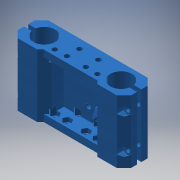
# Autodesk Inventor part: ChimeraXCarriage6
Saved by Autodesk Inventor 2016 (Build 200138000, 138)
## iProperties
Category: Print
Created: 2015-03-10
Part Number: ChimeraXCarriage6
Material: ABS Plastic
Document SubType Name: Modeling
Designer: Jack
Density: 1.06 g/cm^3
Appearance: Cyan
Mass: 40.4192 g
Surface Area: 204.208 cm^2
Volume: 38.1313 cm^3
Author: Jack
Title: Chimera X Carriage V6
Autodesk Inventor part; units mm, degrees
ref_plane "YZ Plane" through (0, 0, 0) normal (1, 0, 0) x (0, 1, 0)
ref_plane "XZ Plane" through (0, 0, 0) normal (0, 1, 0) x (-1, 0, 0)
ref_plane "XY Plane" through (0, 0, 0) normal (0, 0, 1) x (1, 0, 0)
sketch "Sketch1" plane through (0, 0, 0) normal (0, 0, 1) x (1, 0, 0)
  arc A0 (-7.6035, -1.5) -> (-7.6035, 1.5) centre (0, 0) ccw
  arc A1 (62.6035, 1.5) -> (62.6035, -1.5) centre (55, 0) ccw
  line L0 (-7.6035, -1.5) -> (-13, -1.5)
  line L1 (-13, -1.5) -> (-13, -11)
  line L2 (-13, -11) -> (11, -11)
  line L3 (11, -11) -> (11, 3)
  line L4 (11, 3) -> (44, 3)
  line L5 (44, 3) -> (44, -11)
  line L6 (44, -11) -> (68, -11)
  line L7 (68, -11) -> (68, -1.5)
  line L8 (68, -1.5) -> (62.6035, -1.5)
  line L9 (62.6035, 1.5) -> (68, 1.5)
  line L10 (68, 1.5) -> (68, 11)
  line L11 (68, 11) -> (44, 11)
  line L12 (44, 11) -> (44, 11)
  line L13 (44, 11) -> (11, 11)
  line L14 (11, 11) -> (11, 11)
  line L15 (11, 11) -> (-13, 11)
  line L16 (-13, 11) -> (-13, 1.5)
  line L17 (-13, 1.5) -> (-7.6035, 1.5)
  dimension "d0" = 15.5
  dimension "d1" = 55
  dimension "d2" = 1.5
  dimension "d3" = 13
  dimension "d4" = 11
  dimension "d5" = 11
  dimension "d6" = 11
  dimension "d7" = 13
  dimension "d8" = 14
  dimension "d9" = 8
  constraints: 36 end point, 12 perpendicular, 6 point on line, 4 equal length, 4 point on circle, 4 vertical alignment, 2 centre point, 1 coincident, 1 equal radius, 1 horizontal, 1 horizontal alignment, 1 parallel, 1 vertical
  measures "d0" diameter of A0
  measures "d1" distance of A1.centre point (0, 0)
  measures "d2" distance from line of point (0, 0) L0
  measures "d3" distance from line of point (0, 0) L16
  measures "d4" distance from line of L15 point (0, 0)
  measures "d5" distance from line of L14 point (0, 0)
  measures "d6" distance from line of L2 point (0, 0)
  measures "d7" distance from line of A1.centre L10
  measures "d8" distance of L2.end L3.end
  measures "d9" distance between parallel lines of L4 L13
extrude "Extrusion1" add sketch "Sketch1" along normal blind 45
chamfer "Chamfer1" distance 5 angle 45 6 edges at (-13, 11, 22.5) (-13, -11, 22.5) (68, -11, 22.5) (68, 11, 22.5) (44, -11, 22.5) (11, -11, 22.5)
sketch "Sketch2" plane through (-8, 11, 0) normal (0, 1, 0) x (1, 0, 0)
  line L0 (71, 0) -> (71, -45) projected
  line L1 (0, -45) -> (0, 0) projected
  line L2 (76, -45) -> (76, 0) projected
  line L3 (-5, 0) -> (-5, -45) projected
  line L4 (76, 0) -> (71, 0) projected
  line L5 (71, -45) -> (76, -45) projected
  point P0 (8, 0)
  point P1 (-2.5, -10)
  point P2 (-2.5, -35)
  point P3 (73.5, -10)
  point P4 (73.5, -35)
  dimension "d18" = 2.5
  dimension "d19" = 2.5
  dimension "d20" = 10
  dimension "d21" = 10
  constraints: 2 horizontal alignment, 2 vertical alignment
  measures "d18" distance from line of L1 point (-2.5, -10)
  measures "d19" distance from line of L0 point (73.5, -10)
  measures "d20" distance from line of L4 point (73.5, -10)
  measures "d21" distance from line of L5 point (73.5, -35)
hole "Hole1" at (-10.5, 11, 10) at (-10.5, 11, 35) at (65.5, 11, 10) at (65.5, 11, 35) direction (0, -1, 0) diameter 3.5 end through all counterbore diameter 7.3 counterbore depth 5
sketch "Sketch3" plane through (49, -11, 0) normal (0, -1, 0) x (1, 0, 0)
  circle A0 centre (16.5, 10) radius 1.75 projected
  circle A1 centre (16.5, 35) radius 1.75 projected
  circle A2 centre (-59.5, 35) radius 1.75 projected
  circle A3 centre (-59.5, 10) radius 1.75 projected
  line L0 (16.5, 13.1754) -> (19.25, 11.5877)
  line L1 (19.25, 11.5877) -> (19.25, 8.4123)
  line L2 (19.25, 8.4123) -> (16.5, 6.8246)
  line L3 (16.5, 6.8246) -> (13.75, 8.4123)
  line L4 (13.75, 8.4123) -> (13.75, 11.5877)
  line L5 (13.75, 11.5877) -> (16.5, 13.1754)
  line L6 (16.5, 31.8246) -> (13.75, 33.4123)
  line L7 (13.75, 33.4123) -> (13.75, 36.5877)
  line L8 (13.75, 36.5877) -> (16.5, 38.1754)
  line L9 (16.5, 38.1754) -> (19.25, 36.5877)
  line L10 (19.25, 36.5877) -> (19.25, 33.4123)
  line L11 (19.25, 33.4123) -> (16.5, 31.8246)
  circle A4 centre (-59.5, 10) radius 1.75 projected
  line L12 (-59.5, 6.8246) -> (-62.25, 8.4123)
  line L13 (-62.25, 8.4123) -> (-62.25, 11.5877)
  line L14 (-62.25, 11.5877) -> (-59.5, 13.1754)
  line L15 (-59.5, 13.1754) -> (-56.75, 11.5877)
  line L16 (-56.75, 11.5877) -> (-56.75, 8.4123)
  line L17 (-56.75, 8.4123) -> (-59.5, 6.8246)
  line L18 (-59.5, 38.1754) -> (-56.75, 36.5877)
  line L19 (-56.75, 36.5877) -> (-56.75, 33.4123)
  line L20 (-56.75, 33.4123) -> (-59.5, 31.8246)
  line L21 (-59.5, 31.8246) -> (-62.25, 33.4123)
  line L22 (-62.25, 33.4123) -> (-62.25, 36.5877)
  line L23 (-62.25, 36.5877) -> (-59.5, 38.1754)
  point P0 (-49, 0)
  dimension "d29" = 5.5
  constraints: 48 end point, 4 coincident, 4 vertical, 3 parallel, 52 other
  measures "d29" distance between parallel lines of L4 L1
extrude "Extrusion2" cut sketch "Sketch3" against normal blind 5
sketch "Sketch5" plane through (-8, 11, 0) normal (0, 1, 0) x (1, 0, 0)
  line L0 (0, 0) -> (71, 0) projected
  line L1 (52, 0) -> (52, -45) projected
  point P0 (8, 0)
  point P1 (48.5, -22.5)
  point P2 (36.5, -31)
  point P3 (36.5, -14)
  dimension "d44" = 17
  dimension "d45" = 12
  dimension "d46" = 3.5
  dimension "d47" = 22.5
  dimension "d48" = 8.5
  constraints: 1 vertical alignment
  measures "d44" distance of point (36.5, -31) point (36.5, -14)
  measures "d45" horizontal distance of point (36.5, -14) point (48.5, -22.5)
  measures "d46" distance from line of L1 point (48.5, -22.5)
  measures "d47" distance from line of L0 point (48.5, -22.5)
  measures "d48" vertical distance of point (48.5, -22.5) point (36.5, -31)
hole "Hole3" at (40.5, 11, 22.5) at (28.5, 11, 31) at (28.5, 11, 14) direction (0, -1, 0) diameter 3.5 end through all counterbore diameter 7.3 counterbore depth 3.5
sketch "Sketch6" plane through (-8, 11, 0) normal (0, 1, 0) x (1, 0, 0)
  circle A0 centre (48.5, -22.5) radius 3.65 projected
  arc A1 (51.9105, -7.1631) -> (49.5, -4) centre (49.5, -6.5) ccw
  arc A2 (49.5, -41) -> (51.9105, -37.8369) centre (49.5, -38.5) ccw
  arc A3 (49.8388, -30.3064) -> (41.1612, -30.3064) centre (45.5, -31.5) ccw
  arc A4 (41.1612, -14.6936) -> (49.8388, -14.6936) centre (45.5, -13.5) ccw
  arc A5 (41.5, -4) -> (39.0895, -7.1631) centre (41.5, -6.5) ccw
  arc A6 (39.0895, -37.8369) -> (41.5, -41) centre (41.5, -38.5) ccw
  line L0 (41.5, -4) -> (49.5, -4)
  line L1 (51.9105, -7.1631) -> (49.8388, -14.6936)
  line L2 (39.0895, -7.1631) -> (41.1612, -14.6936)
  line L3 (49.8388, -30.3064) -> (51.9105, -37.8369)
  line L4 (41.1612, -30.3064) -> (39.0895, -37.8369)
  line L5 (41.5, -41) -> (49.5, -41)
  point P0 (8, 0)
  dimension "d136" = 9
  dimension "d138" = 4
  dimension "d139" = 9
  dimension "d140" = 9
  dimension "d141" = 18
  dimension "d142" = 3
  dimension "d143" = 7
  dimension "d144" = 7
  dimension "d145" = 5
  dimension "d146" = 4
  constraints: 12 end point, 12 point on circle, 12 tangent, 6 centre point, 3 equal radius, 3 vertical alignment, 2 horizontal alignment, 1 horizontal
  measures "d136" diameter of A3
  measures "d138" horizontal distance of A2.centre A3.centre
  measures "d139" vertical distance of A0.centre A3.centre
  measures "d140" diameter of A4
  measures "d141" distance of A3.centre A4.centre
  measures "d142" horizontal distance of A0.centre A4.centre
  measures "d143" vertical distance of A2.centre A3.centre
  measures "d144" vertical distance of A4.centre A1.centre
  measures "d145" diameter of A1
  measures "d146" horizontal distance of A4.centre A5.centre
extrude "Extrusion3" cut sketch "Sketch6" against normal up to surface (8 mm away) contours L1 A4 L2 A5 L0 A1 | L5 A6 L4 A3 L3 A2
sketch "Sketch7" plane through (0, 0, 45) normal (0, 0, 1) x (1, 0, 0)
  line L0 (11, -6) -> (6, -11) projected
  line L1 (11, -6) -> (11, 3) projected
  line L2 (11, 3) -> (44, 3) projected
  line L3 (44, 3) -> (44, -6) projected
  arc A0 (62.6035, 1.5) -> (62.6035, -1.5) centre (55, 0) ccw projected
  line L4 (8.3, -8.7) -> (46.7, -8.7)
  line L5 (44, -6) -> (49, -11) projected
  dimension "d66" = 8.7
  constraints: 2 end point, 2 point on line, 1 horizontal
  measures "d66" distance from line of A0.centre L4
extrude "Extrusion4" add sketch "Sketch7" against normal blind 5
sketch "Sketch8" plane through (0, 0, 0) normal (0, 0, -1) x (-1, 0, 0)
  line L0 (-11, -6) -> (-8.3, -8.7) projected
  line L1 (-11, 3) -> (-11, -6) projected
  line L2 (-31.5, 3) -> (-11, 3) projected
  line L3 (-44, -6) -> (-44, 3) projected
  line L4 (-46.7, -8.7) -> (-44, -6) projected
  line L5 (-46.7, -8.7) -> (-8.3, -8.7) projected
  line L6 (-31.5, 3) -> (-43.5, 3) projected
  line L7 (-44, 3) -> (-43.5, 3) projected
extrude "Extrusion5" add sketch "Sketch8" against normal blind 5
sketch "Sketch9" plane through (0, 0, 0) normal (0, 0, -1) x (-1, 0, 0)
  arc A0 (7.6035, 1.5) -> (7.6035, -1.5) centre (0, 0) ccw projected
  line L0 (13, 1.5) -> (13, 6) projected
  circle A1 centre (-34.25, 4.45) radius 1.75
  circle A2 centre (-34.25, -4.45) radius 1.75
  circle A3 centre (-20.75, 4.45) radius 1.75
  circle A4 centre (-20.75, -4.45) radius 1.75
  dimension "d71" = 3.5
  dimension "d72" = 13.5
  dimension "d73" = 8.9
  dimension "d74" = 4.45
  dimension "d76" = 33.75
  constraints: 4 centre point, 3 equal radius, 2 horizontal alignment, 2 vertical alignment
  measures "d71" diameter of A1
  measures "d72" distance of A3.centre A1.centre
  measures "d73" distance of A3.centre A4.centre
  measures "d74" vertical distance of A0.centre A3.centre
  measures "d76" distance from line of L0 A3.centre
extrude "Extrusion6" cut sketch "Sketch9" against normal up to surface (5 mm away)
sketch "Sketch10" plane through (0, 0, 45) normal (0, 0, 1) x (1, 0, 0)
  circle A0 centre (34.25, -4.45) radius 1.75 projected
  circle A1 centre (20.75, -4.45) radius 1.75 projected
  arc A2 (19.7702, 3) -> (21.7298, 3) centre (20.75, 4.45) ccw projected
  arc A3 (33.2702, 3) -> (35.2298, 3) centre (34.25, 4.45) ccw projected
  circle A4 centre (20.75, 4.45) radius 1.75 projected
  circle A5 centre (34.25, 4.45) radius 1.75 projected
extrude "Extrusion7" cut sketch "Sketch10" against normal up to surface (5 mm away)
sketch "Sketch11" plane through (0, 0, 40) normal (0, 0, -1) x (-1, 0, 0)
  arc A0 (-21.7298, 3) -> (-19.7702, 3) centre (-20.75, 4.45) ccw projected
  arc A1 (-35.2298, 3) -> (-33.2702, 3) centre (-34.25, 4.45) ccw projected
  circle A2 centre (-20.75, -4.45) radius 1.75 projected
  circle A3 centre (-34.25, -4.45) radius 1.75 projected
  line L0 (-31.0746, 4.45) -> (-32.6623, 1.7)
  line L1 (-32.6623, 1.7) -> (-35.8377, 1.7)
  line L2 (-35.8377, 1.7) -> (-37.4254, 4.45)
  line L3 (-37.4254, 4.45) -> (-35.8377, 7.2)
  line L4 (-35.8377, 7.2) -> (-32.6623, 7.2)
  line L5 (-32.6623, 7.2) -> (-31.0746, 4.45)
  line L6 (-31.0746, -4.45) -> (-32.6623, -7.2)
  line L7 (-32.6623, -7.2) -> (-35.8377, -7.2)
  line L8 (-35.8377, -7.2) -> (-37.4254, -4.45)
  line L9 (-37.4254, -4.45) -> (-35.8377, -1.7)
  line L10 (-35.8377, -1.7) -> (-32.6623, -1.7)
  line L11 (-32.6623, -1.7) -> (-31.0746, -4.45)
  line L12 (-23.9254, -4.45) -> (-22.3377, -1.7)
  line L13 (-22.3377, -1.7) -> (-19.1623, -1.7)
  line L14 (-19.1623, -1.7) -> (-17.5746, -4.45)
  line L15 (-17.5746, -4.45) -> (-19.1623, -7.2)
  line L16 (-19.1623, -7.2) -> (-22.3377, -7.2)
  line L17 (-22.3377, -7.2) -> (-23.9254, -4.45)
  line L18 (-23.9254, 4.45) -> (-22.3377, 7.2)
  line L19 (-22.3377, 7.2) -> (-19.1623, 7.2)
  line L20 (-19.1623, 7.2) -> (-17.5746, 4.45)
  line L21 (-17.5746, 4.45) -> (-19.1623, 1.7)
  line L22 (-19.1623, 1.7) -> (-22.3377, 1.7)
  line L23 (-22.3377, 1.7) -> (-23.9254, 4.45)
  point P0 (0, 0)
  dimension "d81" = 5.5
  constraints: 48 end point, 4 coincident, 4 horizontal, 3 equal length, 52 other
  measures "d81" distance between parallel lines of L8 L11
extrude "Extrusion8" cut sketch "Sketch11" along normal blind 3.5 and the other way blind 3
sketch "Sketch12" plane through (0, 0, 5) normal (0, 0, 1) x (1, 0, 0)
  circle A0 centre (34.25, 4.45) radius 1.75 projected
  line L0 (31.0746, 4.45) -> (32.6623, 1.7) projected
  line L1 (32.6623, 7.2) -> (31.0746, 4.45) projected
  line L2 (35.8377, 7.2) -> (32.6623, 7.2) projected
  line L3 (37.4254, 4.45) -> (35.8377, 7.2) projected
  line L4 (35.8377, 1.7) -> (37.4254, 4.45) projected
  line L5 (32.6623, 1.7) -> (35.8377, 1.7) projected
  circle A1 centre (34.25, -4.45) radius 1.75 projected
  line L6 (31.0746, -4.45) -> (32.6623, -7.2) projected
  line L7 (32.6623, -1.7) -> (31.0746, -4.45) projected
  line L8 (35.8377, -1.7) -> (32.6623, -1.7) projected
  line L9 (37.4254, -4.45) -> (35.8377, -1.7) projected
  line L10 (35.8377, -7.2) -> (37.4254, -4.45) projected
  line L11 (32.6623, -7.2) -> (35.8377, -7.2) projected
  circle A2 centre (20.75, 4.45) radius 1.75 projected
  line L12 (23.9254, 4.45) -> (22.3377, 7.2) projected
  line L13 (22.3377, 1.7) -> (23.9254, 4.45) projected
  line L14 (19.1623, 1.7) -> (22.3377, 1.7) projected
  line L15 (17.5746, 4.45) -> (19.1623, 1.7) projected
  line L16 (19.1623, 7.2) -> (17.5746, 4.45) projected
  line L17 (22.3377, 7.2) -> (19.1623, 7.2) projected
  circle A3 centre (20.75, -4.45) radius 1.75 projected
  line L18 (23.9254, -4.45) -> (22.3377, -1.7) projected
  line L19 (22.3377, -7.2) -> (23.9254, -4.45) projected
  line L20 (19.1623, -7.2) -> (22.3377, -7.2) projected
  line L21 (17.5746, -4.45) -> (19.1623, -7.2) projected
  line L22 (19.1623, -1.7) -> (17.5746, -4.45) projected
  line L23 (22.3377, -1.7) -> (19.1623, -1.7) projected
  point P0 (0, 0)
extrude "Extrusion9" cut sketch "Sketch12" along normal blind 3.5 and the other way blind 3 contours A0 | L1 L2 L3 L4 L5 L0 | A1 | L7 L8 L9 L10 L11 L6 | A2 | L13 L14 L15 L16 L17 L12 | A3 | L19 L20 L21 L22 L23 L18
ref_plane "Work Plane1" through (0, 0, 2) normal (0, 0, -1) x (-1, 0, 0)
sketch "Sketch15" plane through (0, 0, 2) normal (0, 0, -1) x (-1, 0, 0)
  circle A0 centre (-20.75, 4.45) radius 1.75 projected
  circle A1 centre (-20.75, -4.45) radius 1.75 projected
  circle A2 centre (-34.25, -4.45) radius 1.75 projected
  circle A3 centre (-34.25, 4.45) radius 1.75 projected
  line L0 (-6, -11) -> (-8.3, -8.7) projected
  line L1 (-6, -11) -> (8, -11) projected
  line L2 (13, -6) -> (8, -11) projected
  line L3 (13, -6) -> (13, -1.5) projected
  line L4 (13, -1.5) -> (7.6035, -1.5) projected
  arc A4 (7.6035, 1.5) -> (7.6035, -1.5) centre (0, 0) ccw projected
  line L5 (7.6035, 1.5) -> (13, 1.5) projected
  line L6 (13, 1.5) -> (13, 6) projected
  line L7 (8, 11) -> (13, 6) projected
  line L8 (8, 11) -> (-63, 11) projected
  line L9 (-68, 6) -> (-63, 11) projected
  line L10 (-68, 6) -> (-68, 1.5) projected
  line L11 (-68, 1.5) -> (-62.6035, 1.5) projected
  arc A5 (-62.6035, -1.5) -> (-62.6035, 1.5) centre (-55, 0) ccw projected
  line L12 (-62.6035, -1.5) -> (-68, -1.5) projected
  line L13 (-68, -1.5) -> (-68, -6) projected
  line L14 (-63, -11) -> (-68, -6) projected
  line L15 (-63, -11) -> (-49, -11) projected
  line L16 (-46.7, -8.7) -> (-49, -11) projected
  line L17 (-46.7, -8.7) -> (-8.3, -8.7) projected
  line L18 (8, 11) -> (-63, 11) projected
  line L19 (-40, 11) -> (-40, 21.5)
  line L20 (-40, 21.5) -> (-14, 21.5)
  line L21 (-14, 21.5) -> (-14, 11)
  circle A6 centre (-37, 16) radius 1.75
  circle A7 centre (-18, 16) radius 1.75
  dimension "d103" = 27
  dimension "d104" = 26
  dimension "d105" = 10.5
  dimension "d106" = 3.5
  dimension "d107" = 19
  dimension "d108" = 5.5
  dimension "d109" = 3
  constraints: 6 end point, 3 perpendicular, 2 centre point, 2 point on line, 1 equal radius, 1 horizontal alignment
  measures "d103" distance between parallel lines of L6 L21
  measures "d104" distance of L19.end L20.end
  measures "d105" distance between parallel lines of L8 L20
  measures "d106" diameter of A6
  measures "d107" distance of A7.centre A6.centre
  measures "d108" distance from line of L20 A7.centre
  measures "d109" distance from line of L19 A6.centre
extrude "Extrusion12" add sketch "Sketch15" against normal blind 5 contours L8 L19 L20 L21
chamfer "Chamfer3" distance 2.5 angle 45 1 edges at (35.5253, 11, 7)
sketch "Sketch16" plane through (0, 0, 7) normal (0, 0, 1) x (1, 0, 0)
  circle A0 centre (18, 16) radius 1.75 projected
  circle A1 centre (37, 16) radius 1.75 projected
  line L0 (18, 12.8246) -> (15.25, 14.4123)
  line L1 (15.25, 14.4123) -> (15.25, 17.5877)
  line L2 (15.25, 17.5877) -> (18, 19.1754)
  line L3 (18, 19.1754) -> (20.75, 17.5877)
  line L4 (20.75, 17.5877) -> (20.75, 14.4123)
  line L5 (20.75, 14.4123) -> (18, 12.8246)
  line L6 (37, 12.8246) -> (34.25, 14.4123)
  line L7 (34.25, 14.4123) -> (34.25, 17.5877)
  line L8 (34.25, 17.5877) -> (37, 19.1754)
  line L9 (37, 19.1754) -> (39.75, 17.5877)
  line L10 (39.75, 17.5877) -> (39.75, 14.4123)
  line L11 (39.75, 14.4123) -> (37, 12.8246)
  point P0 (0, 0)
  dimension "d115" = 5.5
  constraints: 24 end point, 2 coincident, 1 horizontal alignment, 1 parallel, 1 vertical, 26 other
  measures "d115" distance between parallel lines of L10 L7
extrude "Extrusion13" cut sketch "Sketch16" against normal blind 3
sketch "Sketch17" plane through (0, 0, 45) normal (0, 0, 1) x (1, 0, 0)
  line L0 (68, -6) -> (68, -1.5) projected
  line L1 (-13, -1.5) -> (-13, -6) projected
  line L2 (8.3, -8.7) -> (46.7, -8.7) projected
  circle A0 centre (12.25, -4.7) radius 1.75
  circle A1 centre (42.75, -4.7) radius 1.75
  dimension "d118" = 3.5
  dimension "d119" = 25.25
  dimension "d120" = 25.25
  dimension "d121" = 4
  constraints: 2 centre point, 1 equal radius, 1 horizontal alignment
  measures "d118" diameter of A0
  measures "d119" distance from line of L0 A1.centre
  measures "d120" distance from line of L1 A0.centre
  measures "d121" distance from line of L2 A1.centre
extrude "Extrusion14" cut sketch "Sketch17" against normal up to surface (5 mm away)
sketch "Sketch18" plane through (0, 0, 0) normal (0, 0, -1) x (-1, 0, 0)
  arc A0 (-44, -3.4753) -> (-44, -5.9247) centre (-42.75, -4.7) ccw projected
  arc A1 (-44, -5.9247) -> (-44, -3.4753) centre (-42.75, -4.7) ccw projected
  circle A2 centre (-42.75, -4.7) radius 1.75 projected
  arc A3 (-11, -3.4753) -> (-11, -5.9247) centre (-12.25, -4.7) ccw projected
  arc A4 (-11, -5.9247) -> (-11, -3.4753) centre (-12.25, -4.7) ccw projected
  circle A5 centre (-12.25, -4.7) radius 1.75 projected
extrude "Extrusion15" cut sketch "Sketch18" against normal up to surface (5 mm away)
sketch "Sketch19" plane through (0, 0, 5) normal (0, 0, 1) x (1, 0, 0)
  arc A0 (44, -3.4753) -> (44, -5.9247) centre (42.75, -4.7) ccw projected
  arc A1 (11, -5.9247) -> (11, -3.4753) centre (12.25, -4.7) ccw projected
  line L0 (15.4254, -4.7) -> (13.8377, -7.45)
  line L1 (13.8377, -7.45) -> (10.6623, -7.45)
  line L2 (10.6623, -7.45) -> (9.0746, -4.7)
  line L3 (9.0746, -4.7) -> (10.6623, -1.95)
  line L4 (10.6623, -1.95) -> (13.8377, -1.95)
  line L5 (13.8377, -1.95) -> (15.4254, -4.7)
  line L6 (39.5746, -4.7) -> (41.1623, -1.95)
  line L7 (41.1623, -1.95) -> (44.3377, -1.95)
  line L8 (44.3377, -1.95) -> (45.9254, -4.7)
  line L9 (45.9254, -4.7) -> (44.3377, -7.45)
  line L10 (44.3377, -7.45) -> (41.1623, -7.45)
  line L11 (41.1623, -7.45) -> (39.5746, -4.7)
  point P0 (0, 0)
  dimension "d126" = 5.5
  constraints: 24 end point, 2 coincident, 2 horizontal, 1 collinear, 26 other
  measures "d126" distance between parallel lines of L1 L4
extrude "Extrusion16" cut sketch "Sketch19" against normal blind 3 and the other way blind 3
sketch "Sketch20" plane through (0, 0, 40) normal (0, 0, -1) x (-1, 0, 0)
  circle A0 centre (-12.25, -4.7) radius 1.75 projected
  line L0 (-15.4254, -4.7) -> (-13.8377, -7.45) projected
  line L1 (-13.8377, -1.95) -> (-15.4254, -4.7) projected
  line L2 (-10.6623, -1.95) -> (-13.8377, -1.95) projected
  line L3 (-9.0746, -4.7) -> (-10.6623, -1.95) projected
  line L4 (-10.6623, -7.45) -> (-9.0746, -4.7) projected
  line L5 (-13.8377, -7.45) -> (-10.6623, -7.45) projected
  circle A1 centre (-42.75, -4.7) radius 1.75 projected
  line L6 (-39.5746, -4.7) -> (-41.1623, -1.95) projected
  line L7 (-41.1623, -7.45) -> (-39.5746, -4.7) projected
  line L8 (-44.3377, -7.45) -> (-41.1623, -7.45) projected
  line L9 (-45.9254, -4.7) -> (-44.3377, -7.45) projected
  line L10 (-44.3377, -1.95) -> (-45.9254, -4.7) projected
  line L11 (-41.1623, -1.95) -> (-44.3377, -1.95) projected
  point P0 (0, 0)
extrude "Extrusion17" cut sketch "Sketch20" along normal blind 3 and the other way blind 3 contours A0 | L1 L2 L3 L4 L5 L0 | A1 | L7 L8 L9 L10 L11 L6
body "Solid1"
